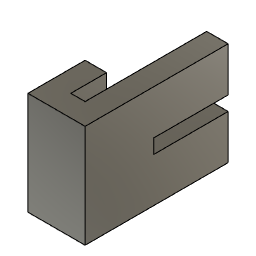
_Switch Extender Holder.05ac75d4-e04a-40db-bbba-b73c21809eca (Autodesk Fusion 360 design; units mm, degrees)
Autodesk Fusion 360 part; units mm, degrees
sketch "Sketch1" plane through (0, 0, 0) normal (0, 0, 1) x (1, 0, 0)
  line L0 (0, 0) -> (7.5, 0)
  line L1 (7.5, 0) -> (7.5, 12.5)
  line L2 (7.5, 12.5) -> (0, 12.5)
  line L3 (0, 12.5) -> (0, 0)
  line L4 (0, 0) -> (12.5, 0)
  line L5 (12.5, 0) -> (12.5, -7.5)
  line L6 (12.5, -7.5) -> (0, -7.5)
  line L7 (0, -7.5) -> (0, 0)
  line L8 (12.5, -7.5) -> (20, -7.5)
  line L9 (20, -7.5) -> (20, 42.5)
  line L10 (20, 42.5) -> (12.5, 42.5)
  line L11 (12.5, 42.5) -> (12.5, -7.5)
  dimension "d1" = 12.5
  dimension "d2" = 50
  dimension "d3" = 7.5
  dimension "d4" = 7.5
  dimension "d5" = 7.5
  dimension "d6" = 12.5
  constraint horizontal L0
  constraint vertical L1
  constraint horizontal L2
  constraint vertical L3
  constraint coincident L0.start L3.end
  constraint horizontal L4
  constraint vertical L5
  constraint horizontal L6
  constraint vertical L7
  constraint horizontal L8
  constraint vertical L9
  constraint horizontal L10
  constraint vertical L11
  measures "d1" distance of L0.start L2.end
  measures "d2" distance of L8.end L9.end
  measures "d3" distance of L1.end L2.end
  measures "d4" distance of L0.start L6.end
  measures "d5" distance of L5.end L8.end
  measures "d6" distance of L0.start L4.end
extrude "Extrude1" add sketch "Sketch1" along normal blind 36
sketch "Sketch2" plane through (20, 0, 0) normal (1, 0, 0) x (0, 1, 0)
  line L0 (-7.5, 36) -> (42.5, 36)
  line L1 (42.5, 36) -> (42.5, 0)
  line L2 (42.5, 0) -> (-7.5, 0)
  line L3 (-7.5, 0) -> (-7.5, 36)
  line L4 (42.5, 20.5) -> (16.5, 20.5)
  line L5 (16.5, 20.5) -> (16.5, 15.5)
  line L6 (16.5, 15.5) -> (42.5, 15.5)
  line L7 (42.5, 15.5) -> (42.5, 20.5)
  dimension "d13" = 15.5
  dimension "d14" = 15.5
  dimension "d16" = 24
  dimension "d17" = 50
  dimension "d19" = 36
  dimension "d21" = 5
  constraint horizontal L0
  constraint vertical L1
  constraint horizontal L2
  constraint vertical L3
  constraint horizontal L4
  constraint vertical L5
  constraint horizontal L6
  constraint vertical L7
  constraint coincident L1 L4.start
  measures "d13" distance of L0.end L4.start
  measures "d14" distance of L1.end L6.end
  measures "d16" distance of L3 L4.end
  measures "d17" distance of L1.end L2.end
  measures "d19" distance of L0.start L2.end
  measures "d21" distance of L4.end L5.end
extrude "Extrude2" cut sketch "Sketch2" along normal through all and the other way through all contours L1 L4 L5 L6 L7
